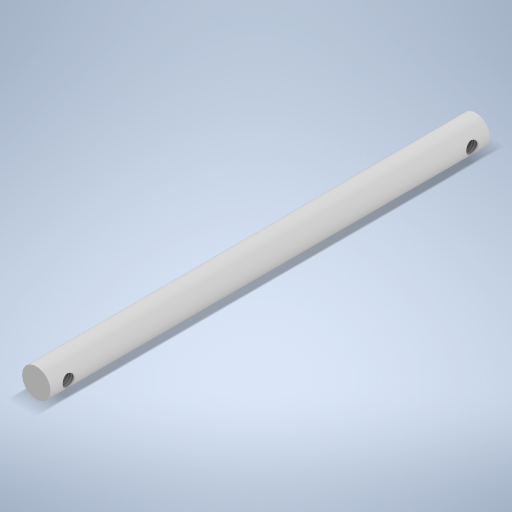
# Autodesk Inventor part: as1
Saved by Autodesk Inventor 2023.2 (Build 272271000, 271)
## iProperties
Created: 2022-12-05
Part Number: as1
Material: Generic
Document SubType Name: Modeling
Designer: daarn
Density: 1 g/cm^3
Appearance: Default
Author: daarn
Autodesk Inventor part; units mm, degrees
ref_plane "YZ Plane" through (0, 0, 0) normal (1, 0, 0) x (0, 1, 0)
ref_plane "XZ Plane" through (0, 0, 0) normal (0, 1, 0) x (-1, 0, 0)
ref_plane "XY Plane" through (0, 0, 0) normal (0, 0, 1) x (1, 0, 0)
sketch "Sketch1" plane through (0, 0, 0) normal (0, 0, 1) x (1, 0, 0)
  circle A0 centre (0, 0) radius 4
  dimension "d0" = 8
  constraints: 1 centre point, 1 coincident
  measures "d0" diameter of A0
extrude "Extrusion1" add sketch "Sketch1" along normal blind 123.051
sketch "Sketch3" plane through (0, 0, 0) normal (1, 0, 0) x (0, 1, 0)
  line L0 (4, 123.051) -> (-4, 123.051) projected
  point P0 (0, 0)
  point P1 (0, 5)
  point P2 (0, 118.051)
  dimension "d14" = 5
  dimension "d15" = 5
  dimension "d16" = 113.051
  constraints: 1 vertical alignment
  measures "d14" distance of point (0, 5) point (0, 0)
  measures "d15" distance from line of L0 point (0, 118.051)
  measures "d16" distance of point (0, 5) point (0, 118.051)
hole "Hole2" at (0, 0, 5) at (0, 0, 118.051) direction (1, 0, 0) diameter 3.242 depth 11.8 thread size "M4x0.7" class "6H" standard "ISO Metric profile"
body "Solid1"
